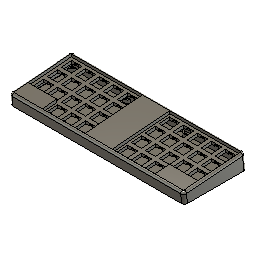
Simple36 Case v48 (Autodesk Fusion 360 design; units mm, degrees)
Autodesk Fusion 360 part; units mm, degrees
note: some values were not read from the file. Set by a fixed rule: which face or edge a step refers to.
sketch "Sketch1" plane through (0, 0, 0) normal (0, 1, 0) x (1, 0, 0)
  line L0 (114.75, 38.25) -> (-114.75, 38.25)
  line L1 (-114.75, 38.25) -> (-114.75, -38.25)
  line L2 (-114.75, -38.25) -> (114.75, -38.25)
  line L3 (114.75, -38.25) -> (114.75, 38.25)
  line L4 (114.75, 38.25) -> (-114.75, -38.25) construction
  line L5 (-114.75, 38.25) -> (114.75, -38.25) construction
  line L6 (111.85, 21.58) -> (97.88, 21.58)
  line L7 (97.88, 21.58) -> (97.88, 35.55)
  line L8 (97.88, 35.55) -> (111.85, 35.55)
  line L9 (111.85, 35.55) -> (111.85, 21.58)
  line L10 (111.85, 21.58) -> (97.88, 35.55) construction
  line L11 (97.88, 21.58) -> (111.85, 35.55) construction
  line L12 (78.83, 21.58) -> (78.83, 35.55)
  line L13 (78.83, 35.55) -> (92.8, 35.55)
  line L14 (92.8, 35.55) -> (92.8, 21.58)
  line L15 (92.8, 21.58) -> (78.83, 21.58)
  line L16 (59.78, 21.58) -> (59.78, 35.55)
  line L17 (59.78, 35.55) -> (73.75, 35.55)
  line L18 (73.75, 35.55) -> (73.75, 21.58)
  line L19 (73.75, 21.58) -> (59.78, 21.58)
  line L20 (40.73, 21.58) -> (40.73, 35.55)
  line L21 (40.73, 35.55) -> (54.7, 35.55)
  line L22 (54.7, 35.55) -> (54.7, 21.58)
  line L23 (54.7, 21.58) -> (40.73, 21.58)
  line L24 (21.68, 21.58) -> (21.68, 35.55)
  line L25 (21.68, 35.55) -> (35.65, 35.55)
  line L26 (35.65, 35.55) -> (35.65, 21.58)
  line L27 (35.65, 21.58) -> (21.68, 21.58)
  line L28 (-35.47, 21.58) -> (-35.47, 35.55)
  line L29 (-35.47, 35.55) -> (-21.5, 35.55)
  line L30 (-21.5, 35.55) -> (-21.5, 21.58)
  line L31 (-21.5, 21.58) -> (-35.47, 21.58)
  line L32 (-54.52, 21.58) -> (-54.52, 35.55)
  line L33 (-54.52, 35.55) -> (-40.55, 35.55)
  line L34 (-40.55, 35.55) -> (-40.55, 21.58)
  line L35 (-40.55, 21.58) -> (-54.52, 21.58)
  line L36 (-73.57, 21.58) -> (-73.57, 35.55)
  line L37 (-73.57, 35.55) -> (-59.6, 35.55)
  line L38 (-59.6, 35.55) -> (-59.6, 21.58)
  line L39 (-59.6, 21.58) -> (-73.57, 21.58)
  line L40 (-92.62, 21.58) -> (-92.62, 35.55)
  line L41 (-92.62, 35.55) -> (-78.65, 35.55)
  line L42 (-78.65, 35.55) -> (-78.65, 21.58)
  line L43 (-78.65, 21.58) -> (-92.62, 21.58)
  line L44 (-111.67, 21.58) -> (-111.67, 35.55)
  line L45 (-111.67, 35.55) -> (-97.7, 35.55)
  line L46 (-97.7, 35.55) -> (-97.7, 21.58)
  line L47 (-97.7, 21.58) -> (-111.67, 21.58)
  line L48 (97.88, 2.53) -> (97.88, 16.5)
  line L49 (97.88, 16.5) -> (111.85, 16.5)
  line L50 (111.85, 16.5) -> (111.85, 2.53)
  line L51 (111.85, 2.53) -> (97.88, 2.53)
  line L52 (78.83, 2.53) -> (78.83, 16.5)
  line L53 (78.83, 16.5) -> (92.8, 16.5)
  line L54 (92.8, 16.5) -> (92.8, 2.53)
  line L55 (92.8, 2.53) -> (78.83, 2.53)
  line L56 (59.78, 2.53) -> (59.78, 16.5)
  line L57 (59.78, 16.5) -> (73.75, 16.5)
  line L58 (73.75, 16.5) -> (73.75, 2.53)
  line L59 (73.75, 2.53) -> (59.78, 2.53)
  line L60 (40.73, 2.53) -> (40.73, 16.5)
  line L61 (40.73, 16.5) -> (54.7, 16.5)
  line L62 (54.7, 16.5) -> (54.7, 2.53)
  line L63 (54.7, 2.53) -> (40.73, 2.53)
  line L64 (21.68, 2.53) -> (21.68, 16.5)
  line L65 (21.68, 16.5) -> (35.65, 16.5)
  line L66 (35.65, 16.5) -> (35.65, 2.53)
  line L67 (35.65, 2.53) -> (21.68, 2.53)
  line L68 (-35.47, 2.53) -> (-35.47, 16.5)
  line L69 (-35.47, 16.5) -> (-21.5, 16.5)
  line L70 (-21.5, 16.5) -> (-21.5, 2.53)
  line L71 (-21.5, 2.53) -> (-35.47, 2.53)
  line L72 (-54.52, 2.53) -> (-54.52, 16.5)
  line L73 (-54.52, 16.5) -> (-40.55, 16.5)
  line L74 (-40.55, 16.5) -> (-40.55, 2.53)
  line L75 (-40.55, 2.53) -> (-54.52, 2.53)
  line L76 (-73.57, 2.53) -> (-73.57, 16.5)
  line L77 (-73.57, 16.5) -> (-59.6, 16.5)
  line L78 (-59.6, 16.5) -> (-59.6, 2.53)
  line L79 (-59.6, 2.53) -> (-73.57, 2.53)
  line L80 (-92.62, 2.53) -> (-92.62, 16.5)
  line L81 (-92.62, 16.5) -> (-78.65, 16.5)
  line L82 (-78.65, 16.5) -> (-78.65, 2.53)
  line L83 (-78.65, 2.53) -> (-92.62, 2.53)
  line L84 (-111.67, 2.53) -> (-111.67, 16.5)
  line L85 (-111.67, 16.5) -> (-97.7, 16.5)
  line L86 (-97.7, 16.5) -> (-97.7, 2.53)
  line L87 (-97.7, 2.53) -> (-111.67, 2.53)
  line L88 (97.88, -16.52) -> (97.88, -2.55)
  line L89 (97.88, -2.55) -> (111.85, -2.55)
  line L90 (111.85, -2.55) -> (111.85, -16.52)
  line L91 (111.85, -16.52) -> (97.88, -16.52)
  line L92 (78.83, -16.52) -> (78.83, -2.55)
  line L93 (78.83, -2.55) -> (92.8, -2.55)
  line L94 (92.8, -2.55) -> (92.8, -16.52)
  line L95 (92.8, -16.52) -> (78.83, -16.52)
  line L96 (59.78, -16.52) -> (59.78, -2.55)
  line L97 (59.78, -2.55) -> (73.75, -2.55)
  line L98 (73.75, -2.55) -> (73.75, -16.52)
  line L99 (73.75, -16.52) -> (59.78, -16.52)
  line L100 (40.73, -16.52) -> (40.73, -2.55)
  line L101 (40.73, -2.55) -> (54.7, -2.55)
  line L102 (54.7, -2.55) -> (54.7, -16.52)
  line L103 (54.7, -16.52) -> (40.73, -16.52)
  line L104 (21.68, -16.52) -> (21.68, -2.55)
  line L105 (21.68, -2.55) -> (35.65, -2.55)
  line L106 (35.65, -2.55) -> (35.65, -16.52)
  line L107 (35.65, -16.52) -> (21.68, -16.52)
  line L108 (-35.47, -16.52) -> (-35.47, -2.55)
  line L109 (-35.47, -2.55) -> (-21.5, -2.55)
  line L110 (-21.5, -2.55) -> (-21.5, -16.52)
  line L111 (-21.5, -16.52) -> (-35.47, -16.52)
  line L112 (-54.52, -16.52) -> (-54.52, -2.55)
  line L113 (-54.52, -2.55) -> (-40.55, -2.55)
  line L114 (-40.55, -2.55) -> (-40.55, -16.52)
  line L115 (-40.55, -16.52) -> (-54.52, -16.52)
  line L116 (-73.57, -16.52) -> (-73.57, -2.55)
  line L117 (-73.57, -2.55) -> (-59.6, -2.55)
  line L118 (-59.6, -2.55) -> (-59.6, -16.52)
  line L119 (-59.6, -16.52) -> (-73.57, -16.52)
  line L120 (-92.62, -16.52) -> (-92.62, -2.55)
  line L121 (-92.62, -2.55) -> (-78.65, -2.55)
  line L122 (-78.65, -2.55) -> (-78.65, -16.52)
  line L123 (-78.65, -16.52) -> (-92.62, -16.52)
  line L124 (-111.67, -16.52) -> (-111.67, -2.55)
  line L125 (-111.67, -2.55) -> (-97.7, -2.55)
  line L126 (-97.7, -2.55) -> (-97.7, -16.52)
  line L127 (-97.7, -16.52) -> (-111.67, -16.52)
  line L128 (59.78, -35.57) -> (59.78, -21.6)
  line L129 (59.78, -21.6) -> (73.75, -21.6)
  line L130 (73.75, -21.6) -> (73.75, -35.57)
  line L131 (73.75, -35.57) -> (59.78, -35.57)
  line L132 (40.73, -35.57) -> (40.73, -21.6)
  line L133 (40.73, -21.6) -> (54.7, -21.6)
  line L134 (54.7, -21.6) -> (54.7, -35.57)
  line L135 (54.7, -35.57) -> (40.73, -35.57)
  line L136 (21.68, -35.57) -> (21.68, -21.6)
  line L137 (21.68, -21.6) -> (35.65, -21.6)
  line L138 (35.65, -21.6) -> (35.65, -35.57)
  line L139 (35.65, -35.57) -> (21.68, -35.57)
  line L140 (-35.47, -35.57) -> (-35.47, -21.6)
  line L141 (-35.47, -21.6) -> (-21.5, -21.6)
  line L142 (-21.5, -21.6) -> (-21.5, -35.57)
  line L143 (-21.5, -35.57) -> (-35.47, -35.57)
  line L144 (-54.52, -35.57) -> (-54.52, -21.6)
  line L145 (-54.52, -21.6) -> (-40.55, -21.6)
  line L146 (-40.55, -21.6) -> (-40.55, -35.57)
  line L147 (-40.55, -35.57) -> (-54.52, -35.57)
  line L148 (-73.57, -35.57) -> (-73.57, -21.6)
  line L149 (-73.57, -21.6) -> (-59.6, -21.6)
  line L150 (-59.6, -21.6) -> (-59.6, -35.57)
  line L151 (-59.6, -35.57) -> (-73.57, -35.57)
  line L152 (-115.75, -39.25) -> (115.75, -39.25)
  line L153 (115.75, -39.25) -> (115.75, 39.25)
  line L154 (115.75, 39.25) -> (-115.75, 39.25)
  line L155 (-115.75, 39.25) -> (-115.75, -39.25)
  line L156 (-118.75, -42.25) -> (118.75, -42.25)
  line L157 (118.75, -42.25) -> (118.75, 42.25)
  line L158 (118.75, 42.25) -> (-118.75, 42.25)
  line L159 (-118.75, 42.25) -> (-118.75, -42.25)
  line L160 (-115.75, -39.25) -> (-76.57, -39.25)
  line L161 (-76.57, -39.25) -> (-76.57, -19.52)
  line L162 (-76.57, -19.52) -> (-115.75, -19.52)
  line L163 (-115.75, -19.52) -> (-115.75, -39.25)
  line L164 (115.75, -39.25) -> (76.75, -39.25)
  line L165 (76.75, -39.25) -> (76.75, -19.52)
  line L166 (76.75, -19.52) -> (115.75, -19.52)
  line L167 (115.75, -19.52) -> (115.75, -39.25)
  line L168 (-18.5, 39.25) -> (18.68, 39.25)
  line L169 (18.68, 39.25) -> (18.68, -39.25)
  line L170 (18.68, -39.25) -> (-18.5, -39.25)
  line L171 (-18.5, -39.25) -> (-18.5, 39.25)
  point P0 (104.865, 28.565)
  dimension "d1" = 229.5
  dimension "d2" = 76.5
  dimension "d4" = 13.97
  dimension "d5" = 2.9
  dimension "d6" = 2.7
  dimension "d9" = -19.05
  dimension "d10" = -19.05
  dimension "d11" = 1
  dimension "d12" = 4
  dimension "d13" = 3
  dimension "d14" = 3
  dimension "d15" = 3
  dimension "d16" = 3
  dimension "d17" = 3
  dimension "d18" = 3
  constraint horizontal L0
  constraint perpendicular L0 L1
  constraint parallel L0 L2
  constraint parallel L1 L3
  constraint coincident L4 origin
  constraint coincident L5 origin
  constraint horizontal L6
  constraint perpendicular L6 L7
  constraint parallel L6 L8
  constraint parallel L7 L9
  constraint coincident L10 P0
  constraint coincident L11 P0
  constraint equal L7 L8
  constraint horizontal L160
  constraint vertical L161
  constraint horizontal L162
  constraint vertical L163
  constraint horizontal L164
  constraint vertical L165
  constraint horizontal L166
  constraint vertical L167
  constraint horizontal L168
  constraint vertical L169
  constraint horizontal L170
  constraint vertical L171
  constraint coincident L152 L169.end
  constraint coincident L154 L168.start
  measures "d1" distance of L1.end L2.end
  measures "d2" distance of L0.end L1.end
  measures "d4" distance of L6.end L7.end
  measures "d5" distance of L3 L9
  measures "d6" distance of L0 L8
  measures "d13" distance of L127 L162
  measures "d14" distance of L148 L161
  measures "d15" distance of L91 L166
  measures "d16" distance of L130 L165
  measures "d17" distance of L104 L169
  measures "d18" distance of L142 L171
extrude "Extrude1" add sketch "Sketch1" along normal blind 4 contours L0 L2 L3 L165 L166 L169 | L0 L3 L153 L154 L166 L169 | L0 L1 L2 L161 L162 L171 | L0 L1 L154 L155 L162 L171 | L2 L152 L165 L169 | L2 L152 L161 L171 makes body 1 at (-57.9067, 0, 26.2567) makes body 2 at (94.4933, 0, 7.2067)
sketch "Sketch2" plane through (0, 0, -35.55) normal (0, 0, 1) x (1, 0, 0)
  line L0 (97.88, 0) -> (111.85, 0)
  line L1 (111.85, 0) -> (111.85, 4)
  line L2 (111.85, 4) -> (97.88, 4)
  line L3 (97.88, 4) -> (97.88, 0)
  line L4 (104.865, 4) -> (104.865, 0) construction
  line L5 (107.365, 0) -> (102.365, 0)
  line L6 (102.365, 0) -> (102.365, 2.7)
  line L7 (102.365, 2.7) -> (107.365, 2.7)
  line L8 (107.365, 2.7) -> (107.365, 0)
  line L9 (107.365, 0) -> (102.365, 2.7) construction
  line L10 (102.365, 0) -> (107.365, 2.7) construction
  point P0 (104.865, 1.35)
  dimension "d21" = 5
  dimension "d23" = 1.3
  constraint midpoint L2 L4.start
  constraint midpoint L0 L4.end
  constraint horizontal L5
  constraint perpendicular L5 L6
  constraint parallel L5 L7
  constraint parallel L6 L8
  constraint coincident L9 P0
  constraint coincident L10 P0
  constraint coincident L4 P0
  constraint coincident L0 L5.start
  measures "d21" distance of L6.end L7.end
  measures "d23" distance of L2 L7
extrude "Extrude2" cut sketch "Sketch2" against normal blind 1 contours L0 L5 L6 L7 L8 bodies 2
extrude "Extrude3" add sketch "Sketch1" along normal blind 4 contours L0 L2 L169 L171 | L0 L154 L168 L169 L171 | L2 L152 L169 L170 L171 bodies 1 2
pattern_linear "R-Pattern1" count 12 spacing 19.05 along (-1, 0, 0) count 4 spacing 19.05 along (0, 0, 1) of "Extrude2"
sketch "Sketch3" plane through (0, 0, -21.58) normal (0, 0, -1) x (-1, 0, 0)
  line L0 (-111.85, 0) -> (-97.88, 0)
  line L1 (-97.88, 0) -> (-97.88, 4)
  line L2 (-97.88, 4) -> (-111.85, 4)
  line L3 (-111.85, 4) -> (-111.85, 0)
  line L4 (-104.865, 4) -> (-104.865, 0) construction
  line L5 (-102.365, 0) -> (-107.365, 0)
  line L6 (-107.365, 0) -> (-107.365, 2.7)
  line L7 (-107.365, 2.7) -> (-102.365, 2.7)
  line L8 (-102.365, 2.7) -> (-102.365, 0)
  line L9 (-102.365, 0) -> (-107.365, 2.7) construction
  line L10 (-107.365, 0) -> (-102.365, 2.7) construction
  point P0 (-104.865, 1.35)
  dimension "d32" = 5
  dimension "d34" = 1.3
  constraint midpoint L2 L4.start
  constraint midpoint L0 L4.end
  constraint horizontal L5
  constraint perpendicular L5 L6
  constraint parallel L5 L7
  constraint parallel L6 L8
  constraint coincident L9 P0
  constraint coincident L10 P0
  constraint coincident L4 P0
  constraint coincident L0 L5.start
  measures "d32" distance of L6.end L7.end
  measures "d34" distance of L2 L7
extrude "Extrude4" cut sketch "Sketch3" against normal blind 1 contours L0 L5 L6 L7 L8 bodies 1
pattern_linear "R-Pattern2" count 4 spacing 19.05 along (0, 0, 1) count 12 spacing 19.05 along (-1, 0, 0) of "Extrude4"
extrude "Extrude5" add sketch "Sketch1" along normal blind 4 contours L0 L2 L169 L171 bodies 1
extrude "Extrude6" add sketch "Sketch1" along normal blind 8 contours L0 L2 L169 L171 | L0 L154 L168 L169 L171 | L2 L3 L152 L153 L164 L165 L166 L167 | L2 L3 L165 L166 | L2 L152 L169 L170 L171 | L1 L2 L161 L162 | L1 L2 L152 L155 L160 L161 L162 L163 | L156 L157 L158 L159 bodies 1
extrude "Extrude7" add sketch "Sketch1" against normal blind 30 contours L156 L157 L158 L159 bodies 1
sketch "Sketch4" plane through (-118.75, 0, 0) normal (-1, 0, 0) x (0, 0, 1)
  line L0 (42.25, -30) -> (42.25, 8)
  line L1 (42.25, 8) -> (-42.25, 8)
  line L2 (-42.25, 8) -> (-42.25, -30)
  line L3 (-42.25, -30) -> (42.25, -30)
  line L4 (-42.25, -14) -> (42.25, -7)
  dimension "d47" = 15
  dimension "d48" = 22
  constraint coincident L2 L4.start
  constraint coincident L0 L4.end
  measures "d47" distance of L0.end L4.end
  measures "d48" distance of L1.end L4.start
extrude "Extrude8" cut sketch "Sketch4" against normal blind 300 contours L0 L2 L3 L4 bodies 1
move_body "Move1" bodies 1 to x (1, 0, 0) y (0, 0.996637, 0.081939) z (0, -0.081939, 0.996637) at (0, 0, 0)
fillet "Fillet1" radius 4 4 edges at (-118.75, -2.9636, 42.1489) (-118.75, 0.472, -42.3537) (118.75, -2.9636, 42.1489) (118.75, 0.472, -42.3537) on bodies 1
fillet "Fillet2" radius 3 8 edges at (117.5784, 4.6072, 41.5958) (118.75, 7.9731, 0.6555) (117.5784, 11.339, -40.2848) (0, 11.435, -41.4524) (-117.5784, 11.339, -40.2848) (-118.75, 7.9731, 0.6555) (-117.5784, 4.6072, 41.5958) (0, 4.5112, 42.7634) on bodies 1
sketch "Sketch5" plane through (0, 3.2161, -39.118) normal (0, -0.081939, 0.996637) x (1, 0, 0)
  line L0 (-115.75, -13.7515) -> (115.75, -13.7515)
  line L1 (115.75, -13.7515) -> (115.75, 0)
  line L2 (115.75, 0) -> (-115.75, 0)
  line L3 (-115.75, 0) -> (-115.75, -13.7515)
  line L4 (0.08, 0) -> (0.08, -13.7515) construction
  line L5 (-115.75, -7.5) -> (115.75, -7.5) construction
  line L6 (-115.75, -4) -> (115.75, -4) construction
  line L7 (5.08, -7.4893) -> (-4.92, -7.4893)
  line L8 (-4.92, -7.4893) -> (-4.92, -3.9893) construction
  line L9 (-4.92, -3.9893) -> (5.08, -3.9893)
  line L10 (5.08, -3.9893) -> (5.08, -7.4893) construction
  line L11 (5.08, -7.4893) -> (-4.92, -3.9893) construction
  line L12 (-4.92, -7.4893) -> (5.08, -3.9893) construction
  line L13 (-3.42, -3.9893) -> (-3.42, -7.4893) construction
  line L14 (0.08, -5.7393) -> (-4.92, -5.7393) construction
  line L15 (0.08, -5.7393) -> (5.08, -5.7393) construction
  arc A0 (-3.42, -3.9893) -> (-3.42, -7.4893) centre (-3.42, -5.7393) ccw
  line L16 (3.58, -4) -> (3.58, -7.5) construction
  arc A1 (3.58, -7.5) -> (3.58, -4) centre (3.58, -5.75) ccw
  line L17 (-3.42, -3.9893) -> (3.58, -4)
  line L18 (3.58, -7.5) -> (-3.42, -7.4893)
  line L19 (12.08, -1.7393) -> (-11.92, -1.7393)
  line L20 (-11.92, -1.7393) -> (-11.92, -9.7393)
  line L21 (-11.92, -9.7393) -> (12.08, -9.7393)
  line L22 (12.08, -9.7393) -> (12.08, -1.7393)
  line L23 (12.08, -1.7393) -> (-11.92, -9.7393) construction
  line L24 (-11.92, -1.7393) -> (12.08, -9.7393) construction
  point P0 (0.08, -5.7393)
  point P1 (0.08, -5.7393)
  dimension "d56" = 115.67
  dimension "d57" = 7.5
  dimension "d58" = 3.5
  dimension "d59" = 10
  dimension "d60" = 3.5
  dimension "d61" = 1.5
  dimension "d62" = 1.5
  dimension "d177" = 24
  dimension "d178" = 8
  constraint coincident L2 L4.start
  constraint coincident L0 L4.end
  constraint perpendicular L0 L4
  constraint coincident L3 L5.start
  constraint coincident L1 L5.end
  constraint perpendicular L1 L5
  constraint coincident L3 L6.start
  constraint coincident L1 L6.end
  constraint perpendicular L1 L6
  constraint horizontal L7
  constraint perpendicular L7 L8
  constraint parallel L7 L9
  constraint parallel L8 L10
  constraint coincident L11 P1
  constraint coincident L12 P1
  constraint coincident L4 P1
  constraint coincident L9 L13.start
  constraint coincident L7 L13.end
  constraint perpendicular L7 L13
  constraint coincident P1 P0
  constraint midpoint L8 L14.end
  constraint midpoint L10 L15.end
  constraint midpoint L13 A0.centre
  constraint coincident L6 L16.start
  constraint coincident L5 L16.end
  constraint perpendicular L7 L16
  constraint midpoint L16 A1.centre
  constraint horizontal L19
  constraint perpendicular L19 L20
  constraint parallel L19 L21
  constraint parallel L20 L22
  constraint coincident L23 P1
  constraint coincident L24 P1
  measures "d56" distance of L1 L4
  measures "d57" distance of L2 L5
  measures "d58" distance of L5 L6
  measures "d59" distance of L8.end L9.end
  measures "d60" distance of L7.end L8.end
  measures "d61" distance of L8 L13
  measures "d62" distance of L10 L16
  measures "d177" distance of L20.end L21.end
  measures "d178" distance of L19.end L20.end
extrude "Extrude9" cut sketch "Sketch5" against normal blind 3 contours L7 A0 A1 L17 bodies 1
sketch "Sketch6" plane through (0, -10.4642, 0.0065) normal (0, -1, 0.000621) x (1, 0, 0)
  ellipse E0 centre (114.75, -39.2479) end of major axis (114.75, -43.2616) minor radius 4 (114.75, -43.2616) -> (118.75, -39.2479) ccw
  line L0 (118.75, -39.2479) -> (118.75, 37.5142)
  ellipse E1 centre (114.75, 37.5142) end of major axis (114.75, 41.5279) minor radius 4 (118.75, 37.5142) -> (114.75, 41.5279) ccw
  line L1 (114.75, 41.5279) -> (-114.75, 41.5279)
  ellipse E2 centre (-114.75, 37.5142) end of major axis (-114.75, 41.5279) minor radius 4 (-114.75, 41.5279) -> (-118.75, 37.5142) ccw
  line L2 (-118.75, 37.5142) -> (-118.75, -39.2479)
  ellipse E3 centre (-114.75, -39.2479) end of major axis (-114.75, -43.2616) minor radius 4 (-118.75, -39.2479) -> (-114.75, -43.2616) ccw
  line L3 (-114.75, -43.2616) -> (114.75, -43.2616)
  line L4 (-115.75, 38.5176) -> (115.75, 38.5176)
  line L5 (115.75, 38.5176) -> (115.75, -40.2513)
  line L6 (115.75, -40.2513) -> (-115.75, -40.2513)
  line L7 (-115.75, -40.2513) -> (-115.75, 38.5176)
  line L8 (-116.75, -41.2513) -> (-116.75, 39.5176)
  line L9 (-116.75, 39.5176) -> (116.75, 39.5176)
  line L10 (116.75, 39.5176) -> (116.75, -41.2513)
  line L11 (116.75, -41.2513) -> (-116.75, -41.2513)
  arc A0 (-115.75, 32.5176) -> (-109.75, 38.5176) centre (-115.75, 38.5176) ccw
  circle A1 centre (-113.75, 36.5176) radius 1.6
  arc A2 (109.75, 38.5176) -> (115.75, 32.5176) centre (115.75, 38.5176) ccw
  circle A3 centre (113.75, 36.5176) radius 1.6
  arc A4 (-5, 38.5176) -> (5, 38.5176) centre (0, 38.5176) ccw
  circle A5 centre (0, 36.5176) radius 1.6
  arc A6 (115.75, -34.2513) -> (109.75, -40.2513) centre (115.75, -40.2513) ccw
  circle A7 centre (113.75, -38.2513) radius 1.6
  arc A8 (-109.75, -40.2513) -> (-115.75, -34.2513) centre (-115.75, -40.2513) ccw
  circle A9 centre (-113.75, -38.2513) radius 1.6
  arc A10 (45.75, -40.2513) -> (35.75, -40.2513) centre (40.75, -40.2513) ccw
  arc A11 (-35.75, -40.2513) -> (-45.75, -40.2513) centre (-40.75, -40.2513) ccw
  circle A12 centre (-40.75, -38.2513) radius 1.6
  circle A13 centre (40.75, -38.2513) radius 1.6
  line L12 (-40.75, -40.2513) -> (-40.75, -35.2513) construction
  line L13 (40.75, -40.2513) -> (40.75, -35.2513) construction
  line L14 (-116.25, 39.0176) -> (116.25, 39.0176)
  line L15 (116.25, 39.0176) -> (116.25, -40.7513)
  line L16 (116.25, -40.7513) -> (-116.25, -40.7513)
  line L17 (-116.25, -40.7513) -> (-116.25, 39.0176)
  dimension "d71" = -1
  dimension "d74" = 6
  dimension "d75" = 3.2
  dimension "d76" = 2
  dimension "d77" = 2
  dimension "d84" = 6
  dimension "d85" = 3.2
  dimension "d86" = 2
  dimension "d87" = 2
  dimension "d94" = 5
  dimension "d95" = 3.2
  dimension "d96" = 2
  dimension "d103" = 6
  dimension "d104" = 3.2
  dimension "d105" = 2
  dimension "d106" = 2
  dimension "d111" = 6
  dimension "d112" = 3.2
  dimension "d113" = 2
  dimension "d114" = 2
  dimension "d123" = 5
  dimension "d124" = 75
  dimension "d125" = 5
  dimension "d126" = 75
  dimension "d127" = 3.2
  dimension "d128" = 2
  dimension "d129" = 3.2
  dimension "d130" = 2
  dimension "d139" = -0.5
  constraint coincident L4.start L7.end
  constraint coincident L5 A2.end
  constraint coincident L4.end L5.start
  constraint midpoint L4 A4.centre
  constraint coincident L5.end L6.start
  constraint coincident L7 A8.end
  constraint coincident L6.end L7.start
  constraint coincident L6 A10.end
  constraint coincident L6 A10.centre
  constraint coincident L6 A11.end
  constraint coincident L6 A11.centre
  constraint coincident A11.centre L12.start
  constraint midpoint A11 L12.end
  constraint perpendicular L6 L12
  constraint coincident A10.centre L13.start
  constraint midpoint A10 L13.end
  constraint perpendicular L6 L13
  constraint coincident A13.centre L13
  measures "d74" radius of A0
  measures "d75" diameter of A1
  measures "d76" distance of L4 A1.centre
  measures "d77" distance of L7 A1.centre
  measures "d84" radius of A2
  measures "d85" diameter of A3
  measures "d86" distance of L4 A3.centre
  measures "d87" distance of L5 A3.centre
  measures "d94" radius of A4
  measures "d95" diameter of A5
  measures "d96" distance of A4.centre A5.centre
  measures "d103" radius of A6
  measures "d104" diameter of A7
  measures "d105" distance of L6 A7.centre
  measures "d106" distance of L5 A7.centre
  measures "d111" radius of A8
  measures "d112" diameter of A9
  measures "d113" distance of L7 A9.centre
  measures "d114" distance of L6 A9.centre
  measures "d123" radius of A10
  measures "d124" distance of L5.end A10.centre
  measures "d125" radius of A11
  measures "d126" distance of L6.end A11.centre
  measures "d127" diameter of A12
  measures "d128" distance of A11.centre A12.centre
  measures "d129" diameter of A13
  measures "d130" distance of L6 A13.centre
fillet "Fillet3" radius 1 4 edges at (5.3273, -2.1725, -42.5712) (0.08, -0.5193, -42.4352) (-5.17, -2.2581, -42.5782) (0.1764, -4.0023, -42.7216) on bodies 1
extrude "Extrude10" cut sketch "Sketch6" against normal blind 3 contours L8 L9 L10 L11 | L14 L15 L16 L17 bodies 1
delete_face "DeleteFace1" 1 faces at (-38.5833, -9.4892, -40.2454) on bodies 1
extrude "Extrude11" add sketch "Sketch6" against normal blind 8 contours L4 L7 A0 bodies 1
extrude "Extrude12" cut sketch "Sketch6" against normal blind 3 contours L4 L7 A0 bodies 1
extrude "Extrude13" add 1 faces at (-113.75, -4.5913, 38.5205) along direction (0, 0.000621, 1) blind 1 on bodies 1 bodies 1
delete_face "DeleteFace2" 1 faces at (-109.75, -4.6077, 38.7199) on bodies 1
extrude "Extrude14" add sketch "Sketch6" against normal blind 8 contours L4 L5 A2 bodies 1
extrude "Extrude15" cut sketch "Sketch6" against normal blind 3 contours L4 L5 A2 bodies 1
extrude "Extrude16" add 1 faces at (113.75, -6.0158, 38.5213) along direction (0, 0.000621, 1) blind 1 on bodies 1 bodies 1
delete_face "DeleteFace3" 1 faces at (109.75, -4.6077, 38.7199) on bodies 1
extrude "Extrude17" add sketch "Sketch6" against normal blind 8 contours L4 A4 bodies 1
extrude "Extrude18" cut sketch "Sketch6" against normal blind 3 contours L4 A4 bodies 1
extrude "Extrude19" add 1 faces at (-1.6667, -4.5913, 38.5205) along direction (0, 0.000621, 1) blind 1 on bodies 1 bodies 1
delete_face "DeleteFace4" 1 faces at (5, -4.6077, 38.8028) on bodies 1
delete_face "DeleteFace5" 1 faces at (-5, -4.6077, 38.8028) on bodies 1
extrude "Extrude20" add sketch "Sketch6" against normal blind 7 contours L5 L6 A6 bodies 1
extrude "Extrude21" cut sketch "Sketch6" against normal blind 3 contours L5 L6 A6 bodies 1
extrude "Extrude22" add sketch "Sketch6" against normal blind 7 contours L6 L7 A8 bodies 1
extrude "Extrude23" cut sketch "Sketch6" against normal blind 3 contours L6 L7 A8 bodies 1
extrude "Extrude24" cut sketch "Sketch6" against normal blind 7 contours A9 bodies 1
extrude "Extrude25" cut sketch "Sketch6" against normal blind 7 contours A7 bodies 1
extrude "Extrude26" add sketch "Sketch6" against normal blind 7 contours L6 A11 | L6 A10 bodies 1
extrude "Extrude27" cut sketch "Sketch6" against normal blind 3 contours L6 A11 | L6 A10 bodies 1
extrude "Extrude28" cut sketch "Sketch6" against normal blind 7 contours A12 bodies 1
extrude "Extrude29" cut sketch "Sketch6" against normal blind 7 contours A13 bodies 1
extrude "Extrude30" add sketch "Sketch6" against normal blind 3 separate body contours L4 L7 A0 | L4 L5 L6 L7 A0 A2 A4 A6 A8 A10 A11 | L4 A4 | L6 L7 A8 | L4 L5 A2 | L6 A11 | L5 L6 A6 | L6 A10 | A1 | A3 | A5 | A7 | A9 | A12 | A13 | L14 L15 L16 L17 makes body 3
hole "Hole1" at (0, -10.4415, 36.5241) direction (0, 1, -0.000621) diameter 2.2 depth 3 tip angle 180 counterbore diameter 3.5 counterbore depth 1.3 bodies 3
hole "Hole2" at (113.75, -10.4415, 36.5241) direction (0, 1, -0.000621) diameter 2.2 depth 3 tip angle 180 counterbore diameter 3.5 counterbore depth 1.3 bodies 3
hole "Hole3" at (113.75, -10.4879, -38.2448) direction (0, 1, -0.000621) diameter 2.2 depth 3 tip angle 180 counterbore diameter 3.5 counterbore depth 1.3 bodies 3
hole "Hole4" at (40.75, -10.4879, -38.2448) direction (0, 1, -0.000621) diameter 2.2 depth 3 tip angle 180 counterbore diameter 3.5 counterbore depth 1.3 bodies 3
hole "Hole5" at (-40.75, -10.4879, -38.2448) direction (0, 1, -0.000621) diameter 2.2 depth 3 tip angle 180 counterbore diameter 3.5 counterbore depth 1.3 bodies 3
hole "Hole6" at (-113.75, -10.4879, -38.2448) direction (0, 1, -0.000621) diameter 2.2 depth 3 tip angle 180 counterbore diameter 3.5 counterbore depth 1.3 bodies 3
hole "Hole7" at (-113.75, -10.4415, 36.5241) direction (0, 1, -0.000621) diameter 2.2 depth 3 tip angle 180 counterbore diameter 3.5 counterbore depth 1.3 bodies 3
extrude "Extrude31" cut sketch "Sketch5" against normal blind 1.5 contours L19 L20 L21 L22 bodies 1
delete_face "DeleteFace6" 1 faces at (-1.0867, -4.1697, -40.7286) on bodies 1
delete_face "DeleteFace7" 1 faces at (3.7301, -4.1703, -40.7287) on bodies 1
named bodies: "Case", "Bottom Plate"
